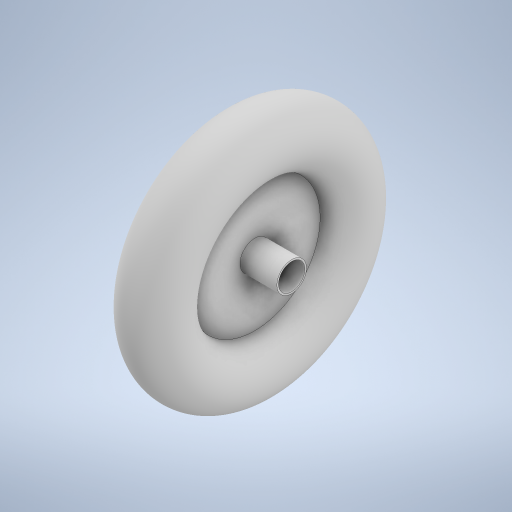
# Autodesk Inventor part: Savior Wheel
Saved by Autodesk Inventor 2024 (Build 280153000, 153)
## iProperties
Created: 2023-12-07
Part Number: Savior Wheel
Material: Generic
Document SubType Name: Modeling
Designer: luke.macenski3281
Density: 1 g/cm^3
Appearance: Default
Author: luke.macenski3281
Autodesk Inventor part; units mm, degrees
ref_plane "YZ Plane" through (0, 0, 0) normal (1, 0, 0) x (0, 1, 0)
ref_plane "XZ Plane" through (0, 0, 0) normal (0, 1, 0) x (-1, 0, 0)
ref_plane "XY Plane" through (0, 0, 0) normal (0, 0, 1) x (1, 0, 0)
sketch "Sketch1" plane through (0, 0, 0) normal (0, 0, 1) x (1, 0, 0)
  line L0 (-23.3654, 0) -> (-10.6654, 0)
  line L1 (-10.6654, 0) -> (-10.6654, 121.92)
  line L2 (-10.6654, 121.92) -> (-23.3654, 121.92)
  line L3 (-23.3654, 121.92) -> (-23.3654, 0)
  circle A0 centre (-17.0154, 121.92) radius 38.1
  point P0 (0, 0)
  point P1 (-10.6654, 84.3529)
  point P2 (-23.3654, 84.3529)
  point P3 (-17.0154, 88.9)
  point P4 (-17.0154, 88.9)
  dimension "d1" = 76.2
  dimension "d2" = 121.92
  dimension "d4" = 12.7
  dimension "d5" = 6.35
  constraints: 8 end point, 2 parallel, 1 centre point, 1 horizontal, 1 midpoint, 1 perpendicular
  measures "d1" diameter of A0
  measures "d2" distance of L2.end L0.start
  measures "d4" distance of L0.start L0.end
  measures "d5" distance of L1.end A0.centre
revolve "Revolution5" add sketch "Sketch1" angle 360 about axis through (-23.3654, 0, 0) along (1, 0, 0)
sketch "Sketch3" plane through (-23.3654, 0, 0) normal (-1, 0, 0) x (0, 0, 1)
  circle A0 centre (0, 0) radius 19.05
  dimension "d10" = 38.1
  constraints: 1 centre point, 1 coincident
  measures "d10" diameter of A0
extrude "Extrusion1" add sketch "Sketch3" along normal blind 25.4
sketch "Sketch4" plane through (-48.7654, 0, 0) normal (-1, 0, 0) x (0, 0, 1)
  circle A0 centre (0, 0) radius 11.1125
  dimension "d13" = 22.225
  constraints: 1 centre point, 1 coincident
  measures "d13" diameter of A0
extrude "Extrusion2" cut sketch "Sketch4" against normal blind 25.4
sketch "Sketch5" plane through (-10.6654, 0, 0) normal (1, 0, 0) x (0, 0, -1)
  circle A0 centre (0, 0) radius 19.05
  circle A1 centre (0, 0) radius 16.891
  dimension "d16" = 38.1
  dimension "d17" = 33.782
  constraints: 2 centre point, 2 coincident
  measures "d16" diameter of A0
  measures "d17" diameter of A1
extrude "Extrusion3" add sketch "Sketch5" along normal blind 47.625
sketch "Sketch6" plane through (-10.6654, 0, 0) normal (1, 0, 0) x (0, 0, -1)
  circle A0 centre (0, 0) radius 11.1125 projected
  circle A1 centre (0, 0) radius 16.891
  point P0 (0, 0)
  constraints: 1 centre point, 1 coincident
extrude "Extrusion4" cut sketch "Sketch6" against normal blind 76.2 contours A0 | A1
body "Solid5"
